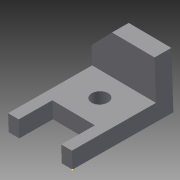
# Autodesk Inventor part: 3-1
Saved by Autodesk Inventor 2015 (Build 190159000, 159)
## iProperties
Created: 2015-09-09
Part Number: 3-1
Material: Generic
Document SubType Name: Modeling
Designer: Brandon
Density: 1 g/cm^3
Appearance: Default
Author: Brandon
Autodesk Inventor part; units mm, degrees
ref_plane "YZ Plane" through (0, 0, 0) normal (1, 0, 0) x (0, 1, 0)
ref_plane "XZ Plane" through (0, 0, 0) normal (0, 1, 0) x (-1, 0, 0)
ref_plane "XY Plane" through (0, 0, 0) normal (0, 0, 1) x (1, 0, 0)
sketch "Sketch1" plane through (0, 0, 0) normal (0, 1, 0) x (-1, 0, 0)
  point P0 (0, 0)
sketch "Sketch2" plane through (0, 0, 0) normal (0, 1, 0) x (-1, 0, 0)
  point P0 (0, 0)
sketch "Sketch3" plane through (0, 0, 0) normal (0, 1, 0) x (-1, 0, 0)
  line L0 (0, 0) -> (76.2, 0)
  line L1 (76.2, 0) -> (76.2, -114.3)
  line L2 (76.2, -114.3) -> (0, -114.3)
  line L3 (0, -114.3) -> (0, 0)
  dimension "d0" = 76.2
  dimension "d1" = 114.3
  constraints: 8 end point, 2 parallel, 1 horizontal, 1 perpendicular
  measures "d0" distance of L1.end L2.end
  measures "d1" distance of L0.end L1.end
extrude "Extrusion1" add sketch "Sketch3" along normal blind 19.05
sketch "Sketch4" plane through (0, 19.05, 0) normal (0, 1, 0) x (1, 0, 0)
  line L0 (-76.2, 0) -> (0, 0) projected
  line L1 (-63.5, 0) -> (-12.7, 0)
  line L2 (-12.7, 0) -> (-12.7, 38.1)
  line L3 (-12.7, 38.1) -> (-63.5, 38.1)
  line L4 (-63.5, 38.1) -> (-63.5, 0)
  dimension "d4" = 12.7
  dimension "d5" = 50.8
  dimension "d6" = 38.1
  constraints: 8 end point, 2 parallel, 1 horizontal, 1 perpendicular, 1 point on line
  measures "d4" distance of L0.start L1.start
  measures "d5" distance of L3.end L2.end
  measures "d6" distance of L1.end L2.end
extrude "Extrusion2" cut sketch "Sketch4" against normal through all
sketch "Sketch5" plane through (0, 19.05, 0) normal (0, 1, 0) x (1, 0, 0)
  line L0 (-76.2, 114.3) -> (0, 114.3)
  line L1 (0, 114.3) -> (0, 95.25)
  line L2 (0, 95.25) -> (-76.2, 95.25)
  line L3 (-76.2, 95.25) -> (-76.2, 114.3)
  point P0 (0, 0)
  dimension "d9" = 76.2
  dimension "d10" = 19.05
  constraints: 8 end point, 2 parallel, 1 horizontal, 1 perpendicular
  measures "d9" distance of L1.end L2.end
  measures "d10" distance of L0.end L1.end
extrude "Extrusion3" add sketch "Sketch5" along normal blind 45.72
sketch "Sketch6" plane through (-76.2, 19.05, -95.25) normal (0, 0, 1) x (1, 0, 0)
  line L0 (0, -19.05) -> (0, 45.72) projected
  line L1 (76.2, 45.72) -> (25.4, 45.72)
  line L2 (0, 45.72) -> (76.2, 45.72) projected
  line L3 (25.4, 45.72) -> (0, 20.32)
  line L4 (0, 20.32) -> (0, 45.72)
  point P0 (76.2, -19.05)
  dimension "d13" = 25.4
  dimension "d15" = 50.8
  constraints: 6 end point, 2 point on line, 1 collinear
  measures "d13" distance of L0.end L3.end
  measures "d15" distance of L1.start L1.end
extrude "Extrusion4" cut sketch "Sketch6" against normal through all
hole "Hole1" at (-38.1, 19.05, -67.818) direction (0, -1, 0) diameter 19.05 end through all
body "Solid1"
